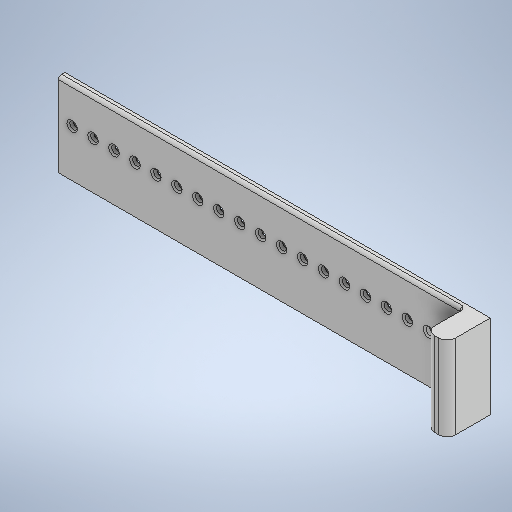
# Autodesk Inventor part: Robot_Front_PushyThingy(TM)
Saved by Autodesk Inventor 2025 (Build 290162010, 162A)
## iProperties
Created: 2024-11-08
Part Number: Robot_Front_PushyThingy(TM)
Material: Generic
Document SubType Name: Modeling
Designer: ishaa
Density: 1 g/cm^3
Appearance: Default
Author: ishaa
Autodesk Inventor part; units mm, degrees
ref_plane "YZ Plane" through (0, 0, 0) normal (1, 0, 0) x (0, 1, 0)
ref_plane "XZ Plane" through (0, 0, 0) normal (0, 1, 0) x (-1, 0, 0)
ref_plane "XY Plane" through (0, 0, 0) normal (0, 0, 1) x (1, 0, 0)
sketch "Sketch1" plane through (0, 0, 0) normal (0, 0, 1) x (1, 0, 0)
  line L0 (-101.5, -20) -> (101.5, -20)
  line L1 (101.5, -20) -> (101.5, 20)
  line L2 (101.5, 20) -> (-101.5, 20)
  line L3 (-101.5, 20) -> (-101.5, -20)
  line L4 (-101.5, -20) -> (101.5, 20) construction
  line L5 (101.5, -20) -> (-101.5, 20) construction
  line L6 (-101.5, 2.5) -> (101.5, 2.5) construction
  circle A0 centre (-95, 2.5) radius 1.75
  circle A1 centre (-85, 2.5) radius 1.75
  circle A2 centre (-75, 2.5) radius 1.75
  circle A3 centre (-65, 2.5) radius 1.75
  circle A4 centre (-55, 2.5) radius 1.75
  circle A5 centre (-45, 2.5) radius 1.75
  circle A6 centre (-35, 2.5) radius 1.75
  circle A7 centre (-25, 2.5) radius 1.75
  circle A8 centre (-15, 2.5) radius 1.75
  circle A9 centre (-5, 2.5) radius 1.75
  circle A10 centre (5, 2.5) radius 1.75
  circle A11 centre (15, 2.5) radius 1.75
  circle A12 centre (25, 2.5) radius 1.75
  circle A13 centre (35, 2.5) radius 1.75
  line L7 (-33.25, 2.5) -> (-26.75, 2.5) construction
  line L8 (0, 28.8941) -> (0, 9.8883) construction
  line L9 (0, -29.7788) -> (0, 38.673) construction
  circle A14 centre (45, 2.5) radius 1.75
  circle A15 centre (55, 2.5) radius 1.75
  circle A16 centre (65, 2.5) radius 1.75
  circle A17 centre (75, 2.5) radius 1.75
  circle A18 centre (85, 2.5) radius 1.75
  circle A19 centre (95, 2.5) radius 1.75
  line L10 (-13.25, 2.5) -> (-6.75, 2.5) construction
  line L11 (-3.25, 2.5) -> (3.25, 2.5) construction
  line L12 (0, 2.5) -> (0, -4.3216) construction
  point P0 (0, 0)
  dimension "d0" = 203
  dimension "d1" = 40
  dimension "d3" = 3.5
  dimension "d6" = 10
  dimension "d64" = 22.5
  constraints: 24 end point, 16 centre point, 5 point on line, 4 horizontal, 4 horizontal alignment, 4 line through centre, 3 midpoint, 2 collinear, 2 parallel, 2 perpendicular, 2 point on circle, 2 vertical, 40 other
  measures "d0" distance of L2.end L1.end
  measures "d1" distance of L1.end L0.end
  measures "d3" diameter of A0
  measures "d6" distance of A0.centre A1.centre
  measures "d64" distance between parallel lines of L0 L6
extrude "Extrusion1" add sketch "Sketch1" along normal blind 3 contours L3 L2 L1 L0 | A19
chamfer "Chamfer1" distance 0.7 angle 45 38 edges at (-66.75, 2.5, 0) (-66.75, 2.5, 3) (-76.75, 2.5, 0) (-86.75, 2.5, 3) (-86.75, 2.5, 0) (-96.75, 2.5, 0) (-96.75, 2.5, 3) (-56.75, 2.5, 0) (-56.75, 2.5, 3) (33.25, 2.5, 0) (33.25, 2.5, 3) (13.25, 2.5, 0) (13.25, 2.5, 3) (-6.75, 2.5, 0) (-6.75, 2.5, 3) (-16.75, 2.5, 3) (-16.75, 2.5, 0) (3.25, 2.5, 3) (3.25, 2.5, 0) (23.25, 2.5, 3) (23.25, 2.5, 0) (-46.75, 2.5, 0) (-46.75, 2.5, 3) (-36.75, 2.5, 0) (-36.75, 2.5, 3) (-26.75, 2.5, 0) (-26.75, 2.5, 3) (-76.75, 2.5, 3) (43.25, 2.5, 0) (43.25, 2.5, 3) (53.25, 2.5, 0) (63.25, 2.5, 3) (63.25, 2.5, 0) (83.25, 2.5, 0) (83.25, 2.5, 3) (53.25, 2.5, 3) (73.25, 2.5, 3) (73.25, 2.5, 0)
sketch "Sketch6" plane through (0, 0, 3) normal (0, 0, 1) x (1, 0, 0)
  line L0 (-101.5, 20) -> (-101.5, -20) projected
  line L1 (-101.5, 20) -> (-91.5, 20)
  line L2 (-91.5, 20) -> (-91.5, -20)
  line L3 (-91.5, -20) -> (-101.5, -20)
  line L4 (-101.5, -20) -> (-101.5, 20)
  circle A0 centre (-95, 2.5) radius 2.45 projected
  line L5 (101.5, 20) -> (-101.5, 20) construction
  line L6 (0, 20) -> (0, -37) construction
  line L7 (101.5, 20) -> (91.5, 20)
  line L8 (91.5, 20) -> (91.5, -20)
  line L9 (91.5, -20) -> (101.5, -20)
  line L10 (101.5, -20) -> (101.5, 20)
  line L11 (-101.5, -20) -> (101.5, -20) projected
  point P0 (0, 0)
  dimension "d55" = 10
  constraints: 18 end point, 4 symmetric about line, 2 collinear, 2 parallel, 1 horizontal, 1 midpoint, 1 perpendicular, 1 point on line, 1 vertical
  measures "d55" distance of L2.end L3.end
extrude "Extrusion5" add sketch "Sketch6" along normal blind 17.5 contours L10 L9 L8 L7
fillet "Fillet6" radius 1.5 2 edges at (-5, 20, 3) (91.5, 0, 3)
fillet "Fillet7" radius 4 2 edges at (91.5, 0, 20.5) (101.5, 0, 20.5)
body "Solid1"
